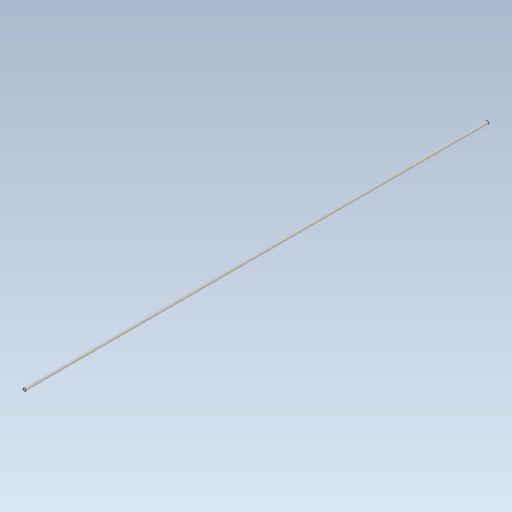
# Autodesk Inventor part: dummyAxis
Saved by Autodesk Inventor 2020 (Build 240168000, 168)
## iProperties
Created: 2019-02-26
Part Number: dummyAxis
Material: Generic
Document SubType Name: Modeling
Designer: LillaHunden
Density: 1 g/cm^3
Appearance: Default
Author: LillaHunden
Autodesk Inventor part; units mm, degrees
ref_plane "YZ Plane" through (0, 0, 0) normal (1, 0, 0) x (0, 1, 0)
ref_plane "XZ Plane" through (0, 0, 0) normal (0, 1, 0) x (-1, 0, 0)
ref_plane "XY Plane" through (0, 0, 0) normal (0, 0, 1) x (1, 0, 0)
sketch "Sketch1" plane through (0, 0, 0) normal (0, 0, 1) x (1, 0, 0)
  circle A0 centre (0, -0.8) radius 0.8 projected
  point P0 (0, 0)
  dimension "d0" = 270.25
  constraints: 1 vertical alignment
extrude "Extrusion1" add sketch "Sketch1" along normal blind 270.25
body "Solid1"
